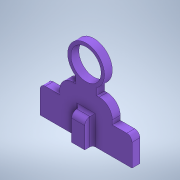
# Autodesk Inventor part: Secondary mount
Saved by Autodesk Inventor 2020 (Build 240168000, 168)
## iProperties
Created: 2021-06-20
Part Number: Secondary mount
Material: Generic
Document SubType Name: Modeling
Designer: ugwue
Density: 1 g/cm^3
Appearance: Violet
Author: ugwue
Autodesk Inventor part; units mm, degrees
ref_plane "YZ Plane" through (0, 0, 0) normal (1, 0, 0) x (0, 1, 0)
ref_plane "XZ Plane" through (0, 0, 0) normal (0, 1, 0) x (-1, 0, 0)
ref_plane "XY Plane" through (0, 0, 0) normal (0, 0, 1) x (1, 0, 0)
sketch "Sketch1" plane through (0, 0, 0) normal (0, 0, 1) x (1, 0, 0)
  circle A0 centre (0, 0) radius 11.5
  arc A1 (20, 0) -> (-20, 0) centre (0, 0) ccw
  line L0 (20, 0) -> (20, -30)
  line L1 (-20, -30) -> (-20, 0)
  line L2 (35, -30) -> (35, -51)
  line L3 (35, -51) -> (-35, -51)
  line L4 (-35, -51) -> (-35, -30)
  line L5 (-35, -30) -> (-20, -30)
  line L6 (20, -30) -> (35, -30)
  constraints: 14 end point, 4 parallel, 2 centre point, 2 coincident, 2 horizontal, 2 perpendicular, 2 point on circle
extrude "Extrusion1" add sketch "Sketch1" along normal blind 6
sketch "Sketch2" plane through (-35, -51, 0) normal (0, -1, 0) x (1, 0, 0)
  line L0 (30, 12) -> (30, -6)
  line L1 (30, -6) -> (40, -6)
  line L2 (40, -6) -> (40, 12)
  line L3 (40, 12) -> (30, 12)
  line L4 (30, 12) -> (40, -6) construction
  line L5 (30, -6) -> (40, 12) construction
  point P0 (35, 0)
  point P1 (35, 3)
  dimension "d7" = 18
  dimension "d8" = 10
  constraints: 12 end point, 2 midpoint, 2 parallel, 1 perpendicular, 1 vertical
  measures "d7" distance of L0.start L0.end
  measures "d8" distance of L1.end L0.end
extrude "Extrusion2" add sketch "Sketch2" against normal blind 20
fillet "Fillet1" radius 2 6 edges at (5, -41, 6) (-5, -41, 6) (5, -41, 0) (-5, -41, 0) (0, -31, 0) (0, -31, 6)
fillet "Fillet2" radius 4 2 edges at (0, -31, 12) (0, -31, -6)
fillet "Fillet3" radius 4 2 edges at (-35, -30, 3) (35, -30, 3)
sketch "Sketch3" plane through (0, 0, 6) normal (0, 0, 1) x (1, 0, 0)
  arc A0 (7.9976, -11.4908) -> (-7.9976, -11.4908) centre (0, 0) ccw
  arc A1 (7.9976, -16.682) -> (-7.9976, -16.682) centre (0, 0) ccw
  line L0 (4, -12.8417) -> (-4, -19.4934) construction
  line L1 (-4, -12.8417) -> (4, -19.4934) construction
  line L2 (-7.9976, -11.4908) -> (-7.9976, -16.682)
  line L3 (7.9976, -11.4908) -> (7.9976, -16.682)
  point P0 (0, -16.1675)
  constraints: 8 end point, 4 point on circle, 2 centre point, 2 coincident, 2 midpoint, 1 parallel, 1 vertical
extrude "Extrusion3" cut sketch "Sketch3" against normal blind 10
sketch "Sketch4" plane through (0, 0, 6) normal (0, 0, 1) x (1, 0, 0)
  line L0 (-7.9976, -11.4908) -> (-7.9976, -16.682) projected
  line L1 (-7.9976, -16.682) -> (-19.8959, -16.682)
  arc A0 (7.9976, -16.682) -> (-7.9976, -16.682) centre (0, 0) ccw projected
  line L2 (7.9976, -16.682) -> (20, -16.682)
  line L3 (20, -30) -> (20, 0) projected
  line L4 (-7.9976, -16.682) -> (-17.0011, 1.4894)
  line L5 (-17.0011, 1.4894) -> (-8.7801, 14.2319)
  line L6 (-8.7801, 14.2319) -> (1.2495, 15.1362)
  line L7 (1.2495, 15.1362) -> (10.7036, 12.5877)
  line L8 (10.7036, 12.5877) -> (15.6744, 3.4985)
  line L9 (15.6744, 3.4985) -> (15.6744, -3.8181)
  line L10 (15.6744, -3.8181) -> (10.5163, -11.3974)
  line L11 (10.5163, -11.3974) -> (8.7045, -14.0594)
  line L12 (8.7045, -14.0594) -> (7.9976, -16.682)
  line L13 (-19.8959, -16.682) -> (-31.3329, 15.1362)
  line L14 (-31.3329, 15.1362) -> (-3.7653, 25.0453)
  line L15 (-3.7653, 25.0453) -> (28.3359, 16.3269)
  line L16 (28.3359, 16.3269) -> (26.8111, -11.3974)
  line L17 (26.8111, -11.3974) -> (20, -16.682)
  constraints: 32 end point, 2 horizontal, 2 perpendicular, 2 point on line, 1 vertical
extrude "Extrusion4" cut sketch "Sketch4" against normal blind 10
sketch "Sketch5" plane through (-19.8959, -16.682, 6) normal (0, 1, 0) x (1, 0, 0)
  line L0 (-7.0101, -7.2709) -> (2.851, -7.2709)
  line L1 (2.851, -7.2709) -> (2.851, 8.3942)
  line L2 (2.851, 8.3942) -> (-7.0101, 8.3942)
  line L3 (-7.0101, 8.3942) -> (-7.0101, -7.2709)
  point P0 (19.8959, 6)
  constraints: 8 end point, 2 parallel, 1 horizontal, 1 perpendicular
extrude "Extrusion5" cut sketch "Sketch5" along normal blind 10
fillet "Fillet4" radius 10 2 edges at (-20, -16.682, 3) (20, -16.682, 3)
body "Solid1"
